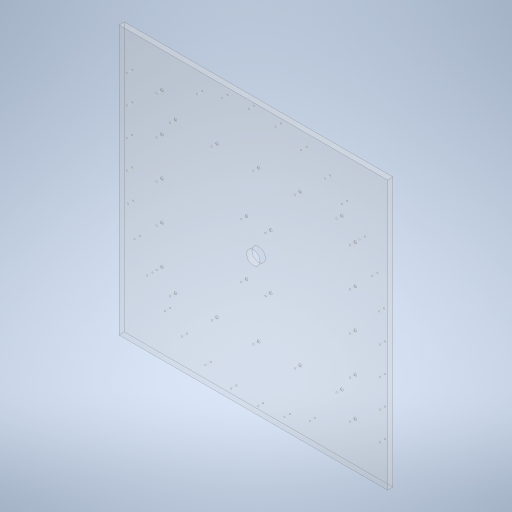
# Autodesk Inventor part: groundPlateWoodV1
Saved by Autodesk Inventor 2024.4 (Build 284460000, 460)
## iProperties
Created: 2025-11-05
Part Number: groundPlateWoodV1
Material: PMMA Plastic
Document SubType Name: Modeling
Designer: jonas
Density: 1.188 g/cm^3
Appearance: Polycarbonate - Clear
Author: jonas
Autodesk Inventor part; units mm, degrees
ref_plane "YZ Plane" through (0, 0, 0) normal (1, 0, 0) x (0, 1, 0)
ref_plane "XZ Plane" through (0, 0, 0) normal (0, 1, 0) x (-1, 0, 0)
ref_plane "XY Plane" through (0, 0, 0) normal (0, 0, 1) x (1, 0, 0)
sketch "Sketch1" plane through (0, 0, 0) normal (0, 1, 0) x (-1, 0, 0)
  line L0 (0, -102.1042) -> (0, 102.1042) construction
  line L1 (37.5532, 0) -> (-37.5532, 0) construction
  line L2 (500, 500) -> (-500, 500)
  line L3 (-500, 500) -> (-500, -500)
  line L4 (-500, -500) -> (500, -500)
  line L5 (500, -500) -> (500, 500)
  circle A0 centre (0, 0) radius 25
  dimension "d0" = 1000
  dimension "d1" = 1000
  dimension "d2" = 50
  constraints: 12 end point, 2 coincident, 2 horizontal, 2 midpoint, 2 parallel, 1 centre point, 1 perpendicular, 1 vertical, 2 other
  measures "d0" distance between parallel lines of L2 L4
  measures "d1" distance between parallel lines of L3 L5
  measures "d2" diameter of A0
extrude "Extrusion1" add sketch "Sketch1" along normal blind 20
sketch "Sketch3" plane through (0, 20, 0) normal (0, 1, 0) x (1, 0, 0)
  line L0 (0, 0) -> (-210, -421.7051) construction
  circle A0 centre (0, 0) radius 25 construction
  line L1 (-116.2595, -456.5292) -> (0, 0) construction
  line L2 (0, 0) -> (-17.2806, -470.783) construction
  line L3 (0, 0) -> (82.477, -463.8241) construction
  line L4 (0, 0) -> (266.5159, -388.4642) construction
  line L5 (329.0291, -337.1573) -> (0, 0) construction
  line L6 (-210, -421.7051) -> (-116.2595, -456.5292) construction
  line L7 (-17.2806, -470.783) -> (-116.2595, -456.5292) construction
  line L8 (-17.2806, -470.783) -> (82.477, -463.8241) construction
  line L9 (82.477, -463.8241) -> (178.5183, -435.9661) construction
  line L10 (178.5183, -435.9661) -> (266.5159, -388.4642) construction
  line L11 (329.0291, -337.1573) -> (395.535, -255.9048) construction
  line L12 (-500, -500) -> (500, -500) construction
  line L13 (0, 0) -> (395.535, -255.9048) construction
  line L14 (395.535, -255.9048) -> (442.392, -161.9398) construction
  line L15 (442.392, -161.9398) -> (0, 0) construction
  line L16 (467.2725, -59.9302) -> (442.392, -161.9398) construction
  line L17 (467.2725, -59.9302) -> (0, 0) construction
  line L18 (471.1, 255) -> (471.1, 150) construction
  line L19 (471.1, 150) -> (471.1, 45) construction
  line L20 (471.1, 360) -> (471.1, 255) construction
  line L21 (500, -500) -> (500, 500) construction
  line L22 (471.1, 45) -> (467.2725, -59.9302) construction
  line L23 (0, 0) -> (178.5183, -435.9661) construction
  line L24 (-178.5183, 435.9661) -> (0, 0) construction
  line L25 (-82.477, 463.8241) -> (0, 0) construction
  line L26 (-82.477, 463.8241) -> (0, 0) construction
  line L27 (17.2806, 470.783) -> (0, 0) construction
  line L28 (116.2595, 456.5292) -> (0, 0) construction
  line L29 (210, 421.7051) -> (0, 0) construction
  line L30 (17.2806, 470.783) -> (-82.477, 463.8241) construction
  line L31 (-82.477, 463.8241) -> (-82.477, 463.8241) construction
  line L32 (-82.477, 463.8241) -> (-178.5183, 435.9661) construction
  line L33 (17.2806, 470.783) -> (116.2595, 456.5292) construction
  line L34 (116.2595, 456.5292) -> (210, 421.7051) construction
  line L35 (-266.5159, 388.4642) -> (-178.5183, 435.9661) construction
  line L36 (-266.5159, 388.4642) -> (0, 0) construction
  line L37 (-395.535, 255.9048) -> (-329.0291, 337.1573) construction
  line L38 (-395.535, 255.9048) -> (-442.392, 161.9398) construction
  line L39 (-471.1, -45) -> (-471.1, -150) construction
  line L40 (-471.1, -150) -> (-471.1, -255) construction
  line L41 (-471.1, -255) -> (-471.1, -360) construction
  line L42 (-329.0291, 337.1573) -> (0, 0) construction
  line L43 (-395.535, 255.9048) -> (0, 0) construction
  line L44 (-442.392, 161.9398) -> (0, 0) construction
  line L45 (-442.392, 161.9398) -> (-467.2725, 59.9302) construction
  line L46 (-467.2725, 59.9302) -> (-471.1, -45) construction
  line L47 (-467.2725, 59.9302) -> (0, 0) construction
  line L48 (-500, 500) -> (-500, -500) construction
  dimension "d20" = 471.1
  dimension "d22" = 210
  dimension "d23" = 100
  dimension "d26" = 105
  dimension "d27" = 28.9
  dimension "d28" = 360
  dimension "d36" = 100
  dimension "d37" = 210
  dimension "d38" = 105
  dimension "d40" = 360
  dimension "d41" = 28.9
  constraints: 92 end point, 40 equal length, 6 vertical alignment, 4 point on line, 2 collinear, 2 perpendicular
  measures "d20" distance of L0.start L0.end
  measures "d22" horizontal distance of L0.end L0.start
  measures "d23" distance of L0.end L1.start
  measures "d26" distance of L5.start L11.end
  measures "d27" distance from line of L21 L20.start
  measures "d28" vertical distance of L0.start L20.start
  measures "d36" distance of L28.start L29.start
  measures "d37" horizontal distance of L0.start L29.start
  measures "d38" distance of L37.start L37.end
  measures "d40" vertical distance of L0.start L41.end
  measures "d41" distance from line of L48 L41.end
hole "Hole2" at (-210, 20, 421.7051) at (-116.2595, 20, 456.5292) at (-17.2806, 20, 470.783) at (82.477, 20, 463.8241) at (178.5183, 20, 435.9661) at (266.5159, 20, 388.4642) at (329.0291, 20, 337.1573) at (395.535, 20, 255.9048) at (442.392, 20, 161.9398) at (467.2725, 20, 59.9302) at (471.1, 20, -45) at (471.1, 20, -150) at (471.1, 20, -255) at (471.1, 20, -360) at (-471.1, 20, 360) at (-471.1, 20, 255) at (-471.1, 20, 150) at (-471.1, 20, 45) at (-467.2725, 20, -59.9302) at (-442.392, 20, -161.9398) at (-395.535, 20, -255.9048) at (-329.0291, 20, -337.1573) at (-266.5159, 20, -388.4642) at (-178.5183, 20, -435.9661) at (-82.477, 20, -463.8241) at (17.2806, 20, -470.783) at (116.2595, 20, -456.5292) at (210, 20, -421.7051) direction (0, -1, 0) diameter 5 end through all
sketch "Sketch4" plane through (0, 20, 0) normal (0, 1, 0) x (1, 0, 0)
  line L0 (500, -500) -> (500, 500) projected
  line L1 (-500, 500) -> (-500, -500) projected
  line L2 (-500, -500) -> (500, -500) projected
  line L3 (500, 500) -> (-500, 500) projected
  line L4 (-360, 220) -> (-360, 77.5) construction
  line L5 (-360, 77.5) -> (-360, -65) construction
  line L6 (-360, -65) -> (-360, -207.5) construction
  line L7 (-360, -207.5) -> (-360, -350) construction
  line L8 (360, 350) -> (360, 207.5) construction
  line L9 (360, 207.5) -> (360, 65) construction
  line L10 (360, 65) -> (360, -77.5) construction
  line L11 (360, -77.5) -> (360, -220) construction
  line L12 (310, -280) -> (155, -280) construction
  line L13 (155, -280) -> (0, -280) construction
  line L14 (0, -280) -> (-155, -280) construction
  line L15 (-155, -280) -> (-310, -280) construction
  line L16 (-310, 280) -> (-155, 280) construction
  line L17 (-155, 280) -> (0, 280) construction
  line L18 (0, 280) -> (155, 280) construction
  line L19 (155, 280) -> (310, 280) construction
  line L20 (0, 7.0345) -> (0, -7.0345) construction
  line L21 (-9.8826, 0) -> (9.8826, 0) construction
  point P0 (0, 0)
  point P1 (-45, 101.5843)
  point P2 (-45, -101.5843)
  point P3 (45, -101.5843)
  point P4 (45, 101.5843)
  point P5 (0, 0)
  dimension "d42" = 140
  dimension "d43" = 140
  dimension "d44" = 150
  dimension "d45" = 150
  dimension "d46" = 570
  dimension "d47" = 570
  dimension "d55" = 220
  dimension "d56" = 220
  dimension "d57" = 50
  dimension "d58" = 50
  dimension "d59" = 90
  constraints: 36 end point, 24 collinear, 12 vertical alignment, 10 horizontal alignment, 3 horizontal, 3 vertical, 2 midpoint, 2 symmetric about line, 1 coincident
  measures "d42" distance from line of L0 L8.start
  measures "d43" distance from line of L1 L7.end
  measures "d44" distance from line of L2 L7.end
  measures "d45" distance from line of L3 L8.start
  measures "d46" distance of L7.end L4.start
  measures "d47" distance of L8.start L11.end
  measures "d55" distance from line of L12.start L2
  measures "d56" vertical distance of L0.end L19.end
  measures "d57" horizontal distance of L11.end L12.start
  measures "d58" horizontal distance of L7.end L15.end
  measures "d59" distance of point (45, 101.584) point (-45, 101.584)
hole "Hole3" at (360, 20, -350) at (360, 20, -207.5) at (360, 20, 77.5) at (360, 20, 220) at (360, 20, -65) at (-360, 20, 350) at (-360, 20, 207.5) at (-360, 20, 65) at (-360, 20, -220) at (-360, 20, -77.5) at (-310, 20, -280) at (-155, 20, -280) at (0, 20, -280) at (155, 20, -280) at (310, 20, -280) at (310, 20, 280) at (155, 20, 280) at (0, 20, 280) at (-155, 20, 280) at (-310, 20, 280) at (-45, 20, -101.5843) at (45, 20, -101.5843) at (-45, 20, 101.5843) at (45, 20, 101.5843) direction (0, -1, 0) diameter 5.5 end through all countersink diameter 10.4 countersink angle 90 clearance for "Countersunk Flat Head Screw DIN EN ISO 2009" size "M5" standard "DIN"
body "Solid1"
